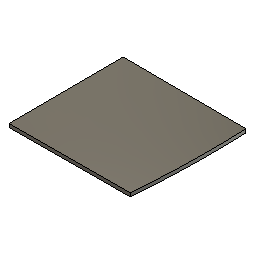
oceaan-25-floor_2 v4 (Autodesk Fusion 360 design; units mm, degrees)
Autodesk Fusion 360 part; units mm, degrees
note: some values were not read from the file. Set by a fixed rule: which sketch regions a step uses.
sketch "Sketch1" plane through (0, 0, 0) normal (0, 1, 0) x (1, 0, 0)
  line L0 (438.1111, -2.1242) -> (11.1168, -4.3194)
  line L1 (9.0295, 401.6753) -> (446.0495, 398.9219)
  line L2 (11.1168, -4.3194) -> (9.0295, 401.6753)
  line L3 (445.4874, 398.9219) -> (446.4173, 398.9267)
  arc A0 (438.1111, -2.1242) -> (446.4173, 398.9267) centre (-2835.5503, 266.2878) ccw
extrude "Extrude1" add sketch "Sketch1" along normal blind 12.5
